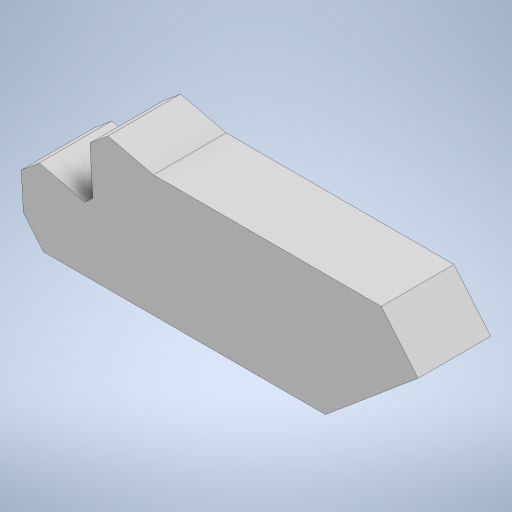
# Autodesk Inventor part: отстойник осветлитель Dummu 2
Saved by Autodesk Inventor 2024.2 (Build 282272000, 272)
## iProperties
Created: 2024-04-06
Part Number: отстойник осветлитель Dummu 2
Material: Generic
Document SubType Name: Modeling
Designer: admin
Density: 1 g/cm^3
Appearance: Default
Author: admin
Autodesk Inventor part; units mm, degrees
ref_plane "YZ Plane" through (0, 0, 0) normal (1, 0, 0) x (0, 1, 0)
ref_plane "XZ Plane" through (0, 0, 0) normal (0, 1, 0) x (-1, 0, 0)
ref_plane "XY Plane" through (0, 0, 0) normal (0, 0, 1) x (1, 0, 0)
sketch "Sketch1" plane through (0, 0, 0) normal (0, 0, 1) x (1, 0, 0)
  line L0 (0, 0) -> (6600, 0)
  line L1 (6600, 0) -> (8767.9058, 1819.0889)
  line L2 (8767.9058, 1819.0889) -> (7906.5704, 2845.5885)
  line L3 (7906.5704, 2845.5885) -> (2576.5704, 2845.5885)
  line L4 (8165.3393, 2537.1997) -> (7533.6745, 2007.1699) construction
  line L5 (7533.6745, 2007.1699) -> (6830.1578, 2845.5885) construction
  line L6 (0, 0) -> (-466.021, 555.3822)
  line L7 (-466.021, 555.3822) -> (-517.5615, 1398.062)
  line L8 (-517.5615, 1398.062) -> (-96.5445, 1751.3372)
  line L9 (-96.5445, 1751.3372) -> (967.9305, 1495.7794)
  line L10 (967.9305, 1495.7794) -> (1157.9095, 1655.1907)
  line L11 (1157.9095, 1655.1907) -> (1091.0783, 2747.8711)
  line L12 (1091.0783, 2747.8711) -> (1512.0954, 3101.1463)
  line L13 (1512.0954, 3101.1463) -> (2576.5704, 2845.5885)
  dimension "d0" = 6600
  dimension "d1" = 2830
  dimension "d2" = 140
  dimension "d3" = 1340
  dimension "d4" = 5330
  dimension "d5" = 725
  dimension "d6" = 73
  dimension "d7" = 73
  dimension "d8" = 880
  dimension "d9" = 248
  dimension "d10" = 73
  constraints: 28 end point, 4 point on line, 3 equal length, 3 perpendicular, 2 horizontal, 2 parallel
  measures "d0" distance of L0.start L0.end
  measures "d1" distance of L0.end L1.end
  measures "d2" angle of L1 L0
  measures "d3" distance of L1.end L2.end
  measures "d4" distance of L2.end L3.end
  measures "d5" distance of L0.start L6.end
  measures "d6" angle of L9 L7
  measures "d7" angle of L13 L11
  measures "d8" distance between parallel lines of L10 L8
  measures "d9" distance of L9.end L10.end
  measures "d10" angle of L11 L9
extrude "Extrusion1" add sketch "Sketch1" along normal mid plane 1700
equation "\"d7\" = d6"
equation "\"d10\" = d6"
body "Solid1"
